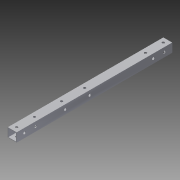
# Autodesk Inventor part: Rebuild Shooter Tower Motor Mount Tube
Saved by Autodesk Inventor 2014 SP1 (Build 180222100, 222)
## iProperties
Created: 2013-10-25
Part Number: Rebuild Shooter Tower Motor Mount Tube
Material: Aluminum 6061
Document SubType Name: Modeling
Designer: Moses
Mass: 178.444 g
Surface Area: 840.674 cm^2
Volume: 65.8466 cm^3
Density: 2.71 g/cm^3
Appearance: Aluminum - Flat
Author: Moses
Autodesk Inventor part; units mm, degrees
ref_plane "YZ Plane" through (0, 0, 0) normal (1, 0, 0) x (0, 1, 0)
ref_plane "XZ Plane" through (0, 0, 0) normal (0, 1, 0) x (-1, 0, 0)
ref_plane "XY Plane" through (0, 0, 0) normal (0, 0, 1) x (1, 0, 0)
sketch "Sketch1" plane through (0, 0, 0) normal (0, 0, 1) x (1, 0, 0)
  line L0 (0, 0) -> (25.4, 0)
  line L1 (25.4, 0) -> (25.4, 25.4)
  line L2 (25.4, 25.4) -> (0, 25.4)
  line L3 (0, 25.4) -> (0, 0)
  line L4 (1.5875, 23.8125) -> (23.8125, 23.8125)
  line L5 (23.8125, 23.8125) -> (23.8125, 1.5875)
  line L6 (23.8125, 1.5875) -> (1.5875, 1.5875)
  line L7 (1.5875, 1.5875) -> (1.5875, 23.8125)
  dimension "d0" = 25.4
  dimension "d1" = 25.4
  dimension "d2" = 1.5875
  constraints: 16 end point, 4 parallel, 2 perpendicular, 1 horizontal, 3 other
  measures "d0" distance of L2.end L1.end
  measures "d1" distance of L1.end L0.end
  measures "d2" distance between parallel lines of L1 L5
extrude "Extrusion1" add sketch "Sketch1" along normal blind 444.5
sketch "Sketch2" plane through (0, 25.4, 0) normal (0, 1, 0) x (1, 0, 0)
  line L0 (25.4, 0) -> (0, 0) projected
  line L1 (25.4, -444.5) -> (0, -444.5) projected
  circle A0 centre (12.7, -381) radius 3.3782 projected
  circle A1 centre (12.7, -431.8) radius 3.3782 projected
  circle A2 centre (13.4937, -237.4032) radius 3.3782 projected
  circle A3 centre (13.4937, -303.4032) radius 3.3782 projected
  line L2 (28.0987, -227.8782) -> (28.0987, -312.9282) construction
  line L3 (0.7937, -312.9282) -> (28.0987, -312.9282) construction
  line L4 (0.7937, -227.8782) -> (0.7937, -312.9282) projected
  line L5 (28.0987, -227.8782) -> (0.7937, -227.8782) construction
  circle A4 centre (12.7, -12.7) radius 3.3782 projected
  circle A5 centre (12.7, -63.5) radius 3.3782 projected
  line L6 (12.7, 0) -> (12.7, -444.5) construction
  constraints: 2 end point, 2 midpoint
extrude "Extrusion2" cut sketch "Sketch2" against normal blind 25.4
sketch "Sketch3" plane through (0, 0, 0) normal (-1, 0, 0) x (0, 0, 1)
  circle A0 centre (422.275, 12.7) radius 3.3782 projected
  circle A1 centre (390.525, 12.7) radius 3.3782 projected
  circle A2 centre (305.6657, 12.7) radius 3.3782 projected
  circle A3 centre (235.8157, 12.7) radius 3.3782 projected
  circle A4 centre (53.975, 12.7) radius 3.3782 projected
  circle A5 centre (22.225, 12.7) radius 3.3782 projected
extrude "Extrusion3" cut sketch "Sketch3" against normal blind 25.4
body "Solid1"
